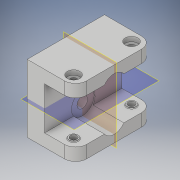
# Autodesk Inventor part: belt_tensioner
Saved by Autodesk Inventor 2019.4 (Build 234330000, 330)
## iProperties
Created: 2020-08-29
Part Number: belt_tensioner
Material: Generisch
Document SubType Name: Modeling
Designer: marc
Density: 1 g/cm^3
Appearance: Vorgabe
Author: marc
## iProperties of the stored document _3D-Druck.ipt
Created: 2020-08-29
Part Number: _3D-Druck
Material: Generisch
Document SubType Name: Modeling
Designer: marc
Density: 1 g/cm^3
Appearance: Vorgabe
Author: marc
Autodesk Inventor part; units mm, degrees
ref_plane "YZ Plane" through (0, 0, 0) normal (1, 0, 0) x (0, 1, 0)
ref_plane "XZ Plane" through (0, 0, 0) normal (0, 1, 0) x (-1, 0, 0)
ref_plane "XY Plane" through (0, 0, 0) normal (0, 0, 1) x (1, 0, 0)
sketch "Skizze1" plane through (0, 0, 0) normal (0, 0, 1) x (1, 0, 0)
  line L0 (0, 0) -> (-25, 0)
  line L1 (-25, 0) -> (-25, 35)
  line L2 (-25, 35) -> (0, 35)
  line L3 (0, 35) -> (0, 0)
  dimension "d0" = 25
  dimension "d1" = 35
  constraints: 8 end point, 2 parallel, 1 horizontal, 1 perpendicular
  measures "d0" distance of L1.end L2.end
  measures "d1" distance of L0.end L1.end
extrude "Extrusion1" add sketch "Skizze1" along normal blind 40
sketch "Skizze2" plane through (0, 0, 40) normal (0, 0, 1) x (1, 0, 0)
  line L0 (0, 6.5) -> (-16, 6.5)
  line L1 (-16, 6.5) -> (-16, 28.5)
  line L2 (-16, 28.5) -> (0, 28.5)
  line L3 (0, 28.5) -> (0, 6.5)
  line L4 (-25, 0) -> (0, 0) projected
  line L5 (0, 35) -> (-25, 35) projected
  line L6 (0, 0) -> (0, 35) projected
  dimension "d4" = 22
  dimension "d5" = 35
  dimension "d6" = 6.5
  dimension "d7" = 16
  constraints: 8 end point, 2 parallel, 1 horizontal, 1 perpendicular, 1 point on line
  measures "d4" distance of L2.end L0.start
  measures "d5" distance between parallel lines of L4 L5
  measures "d6" distance between parallel lines of L5 L2
  measures "d7" distance between parallel lines of L1 L3
extrude "Extrusion2" cut sketch "Skizze2" against normal blind 40
sketch "Skizze3" plane through (0, 0, 40) normal (1, 0, 0) x (0, 0, -1)
  line L0 (0, 6.5) -> (0, 28.5) projected
  line L1 (40, 28.5) -> (40, 6.5) projected
  line L2 (40, 6.5) -> (0, 6.5) projected
  line L3 (40, 35) -> (0, 35) projected
  line L4 (40, 0) -> (0, 0) projected
  point P0 (20, 10)
  point P1 (20, 25)
  dimension "d10" = 15
  dimension "d11" = 20
  dimension "d12" = 40
  dimension "d15" = 35
  dimension "d16" = 10
  constraints: 1 vertical alignment
  measures "d10" distance of point (20, 25) point (20, 10)
  measures "d11" distance from line of L0 point (20, 10)
  measures "d12" distance between parallel lines of L0 L1
  measures "d15" distance between parallel lines of L3 L4
  measures "d16" distance from line of point (20, 10) L4
hole "Bohrung1" at (0, 10, 20) at (0, 25, 20) direction (-1, 0, 0) diameter 5.5 end through all counterbore diameter 12.24 counterbore depth 16.5 clearance for "Sechskantbolzen" size "M5" standard "ANSI Metrisches M Profil"
sketch "Skizze4" plane through (-25, 35, 0) normal (0, 1, 0) x (1, 0, 0)
  line L0 (9, -40) -> (9, 0) projected
  line L1 (9, -40) -> (9, 0) projected
  line L2 (9, -13.88) -> (9, -26.12) projected
  line L3 (25, -40) -> (0, -40) projected
  line L4 (0, 0) -> (25, 0) projected
  point P0 (9, -14.9796)
  point P1 (9, -25.0204)
  point P2 (19, -5)
  point P3 (19, -35)
  dimension "d24" = 5
  dimension "d25" = 5
  dimension "d26" = 10
  constraints: 1 vertical alignment
  measures "d24" distance from line of L3 point (19, -35)
  measures "d25" distance from line of L4 point (19, -5)
  measures "d26" distance from line of L0 point (19, -5)
hole "Bohrung2" at (-6, 35, 5) at (-6, 35, 35) direction (0, -1, 0) diameter 3.4 end through all counterbore diameter 6.5 counterbore depth 2.4 clearance for "Zylinderschraube mit Schlitz DIN 84" size "M3" standard "DIN"
sketch "Skizze5" plane through (-16, 28.5, 40) normal (0, -1, 0) x (1, 0, 0)
  circle A0 centre (10, -5) radius 2.25
  circle A1 centre (10, -5) radius 1.7 projected
  point P0 (16, -40)
  dimension "d34" = 4.5
  constraints: 1 centre point, 1 concentric
  measures "d34" diameter of A0
extrude "Extrusion3" add sketch "Skizze5" along normal blind 0.5
chamfer "Fase1" distance 0.3 angle 45 1 edges at (-8.25, 28.5, 35)
ref_plane "Arbeitsebene1" through (-25, 17.5, 0) normal (0, -1, 0) x (1, 0, 0)
ref_plane "Arbeitsebene2" through (0, 0, 20) normal (0, 0, 1) x (1, 0, 0)
mirror "Spiegeln1" about plane through (0, 0, 20) normal (0, 0, 1) of "Extrusion3", "Fase1"
mirror "Spiegeln2" about plane through (-25, 17.5, 0) normal (0, -1, 0) of "Extrusion3"
chamfer "Fase2" distance 0.3 angle 45 1 edges at (-8.25, 6.5, 35)
mirror "Spiegeln3" about plane through (0, 0, 20) normal (0, 0, 1) of "Extrusion3", "Spiegeln2", "Fase2"
fillet "Rundung1" radius 5.75 4 edges at (0, 3.25, 0) (0, 3.25, 40) (0, 31.75, 40) (0, 31.75, 0)
equation "\"d6\" = -0.5 * d4 + 0.5 * d5"
equation "\"d11\" = 0.5 * d12"
equation "\"d16\" = -0.5 * d10 + 0.5 * d15"
